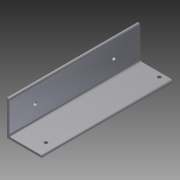
# Autodesk Inventor part: cRIO bracket
Saved by Autodesk Inventor 2012 (Build 160160000, 160)
## iProperties
Created: 2012-05-12
Part Number: cRIO bracket
Material: Default
Document SubType Name: Modeling
Designer: esv
Density: 1 g/cm^3
Author: esv
Autodesk Inventor part; units mm, degrees
ref_plane "YZ Plane" through (0, 0, 0) normal (1, 0, 0) x (0, 1, 0)
ref_plane "XZ Plane" through (0, 0, 0) normal (0, 1, 0) x (-1, 0, 0)
ref_plane "XY Plane" through (0, 0, 0) normal (0, 0, 1) x (1, 0, 0)
sketch "Sketch1" plane through (0, 0, 0) normal (0, 0, 1) x (1, 0, 0)
  line L0 (0, 0) -> (3.175, 0)
  line L1 (3.175, 6.35) -> (3.175, 47.625)
  line L2 (0, 50.8) -> (0, 50.8)
  line L3 (0, 50.8) -> (0, 0)
  line L4 (0, 0) -> (50.8, 0)
  line L5 (50.8, 0) -> (50.8, 0)
  line L6 (47.625, 3.175) -> (6.35, 3.175)
  line L7 (0, 3.175) -> (0, 0)
  arc A0 (3.175, 6.35) -> (6.35, 3.175) centre (6.35, 6.35) ccw
  arc A1 (50.8, 0) -> (47.625, 3.175) centre (47.625, 0) ccw
  arc A2 (3.175, 47.625) -> (0, 50.8) centre (0, 47.625) ccw
  point P0 (3.175, 50.8)
  dimension "d0" = 3.175
  dimension "d1" = 50.8
  dimension "d2" = 3.175
  dimension "d3" = 3.175
  constraints: 16 end point, 6 point on circle, 6 tangent, 4 parallel, 4 perpendicular, 4 point on line, 3 centre point, 2 horizontal, 1 equal radius
  measures "d0" distance of point (3.175, 50.8) L2.end
  measures "d1" distance of L0.start L4.end
  measures "d2" radius of A0
  measures "d3" radius of A1
extrude "Bracket" add sketch "Sketch1" along normal blind 190.5
sketch "Sketch2" plane through (0, 0, 0) normal (-1, 0, 0) x (0, 0, 1)
  line L0 (0, 50.8) -> (190.5, 50.8) projected
  line L1 (0, 50.8) -> (0, 0) projected
  line L2 (0, 0) -> (190.5, 0) projected
  line L3 (38.1, 25.4) -> (152.4, 25.4)
  dimension "d6" = 114.3
  dimension "d7" = 38.1
  dimension "d8" = 25.4
  constraints: 2 end point, 1 parallel
  measures "d6" distance of L3.start L3.end
  measures "d7" distance from line of L1 L3.start
  measures "d8" distance between parallel lines of L0 L3
hole "Mounting Holes" at (0, 25.4, 38.1) at (0, 25.4, 152.4) direction (1, 0, 0) diameter 5.1054 end through all clearance for "Flat Head Machine Screw (82)" size "#10" standard "Ansi Unified Screw Threads"
sketch "Sketch3" plane through (0, 0, 0) normal (0, -1, 0) x (1, 0, 0)
  line L0 (50.8, 190.5) -> (0, 190.5) projected
  line L1 (0, 0) -> (0, 190.5) projected
  line L2 (50.8, 0) -> (50.8, 190.5) projected
  line L3 (37.3062, 171.45) -> (37.3063, 6.35)
  dimension "d16" = 37.3062
  dimension "d17" = 19.05
  dimension "d25" = 165.1
  constraints: 2 end point, 1 parallel
  measures "d16" distance between parallel lines of L1 L3
  measures "d17" distance from line of L0 L3.start
  measures "d25" distance of L3.start L3.end
hole "cRIO Holes" at (37.3062, 0, 171.45) at (37.3063, 0, 6.35) direction (0, 1, 0) diameter 5.1054 end through all clearance for "Flat Head Machine Screw (82)" size "#10" standard "Ansi Unified Screw Threads"
body "Solid1"
